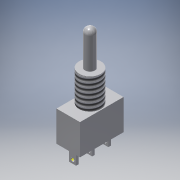
# Autodesk Inventor part: 1MS2
Saved by Autodesk Inventor 2016 (Build 200138000, 138)
## iProperties
Created: 2016-06-17
Part Number: 1MS2
Material: Aluminum
Document SubType Name: Modeling
Designer: Tyler
Density: 2.71 g/cm^3
Appearance: Satin
Author: Tyler
Autodesk Inventor part; units mm, degrees
ref_plane "YZ Plane" through (0, 0, 0) normal (1, 0, 0) x (0, 1, 0)
ref_plane "XZ Plane" through (0, 0, 0) normal (0, 1, 0) x (-1, 0, 0)
ref_plane "XY Plane" through (0, 0, 0) normal (0, 0, 1) x (1, 0, 0)
sketch "Sketch1" plane through (0, 0, 0) normal (0, 0, 1) x (1, 0, 0)
  line L0 (-3.43, -6.35) -> (3.43, -6.35)
  line L1 (3.43, -6.35) -> (3.43, 6.35)
  line L2 (3.43, 6.35) -> (-3.43, 6.35)
  line L3 (-3.43, 6.35) -> (-3.43, -6.35)
  line L4 (-3.43, -6.35) -> (3.43, 6.35) construction
  line L5 (3.43, -6.35) -> (-3.43, 6.35) construction
  point P0 (0, 0)
  dimension "d0" = 6.86
  dimension "d1" = 12.7
  constraints: 12 end point, 2 midpoint, 2 parallel, 1 horizontal, 1 perpendicular
  measures "d0" distance of L2.end L1.end
  measures "d1" distance of L1.end L0.end
extrude "Extrusion1" add sketch "Sketch1" against normal blind 8.89
sketch "Sketch2" plane through (0, 0, 0) normal (0, 0, 1) x (1, 0, 0)
  circle A0 centre (0, 0) radius 3.175
  dimension "d35" = 6.35
  constraints: 1 centre point, 1 coincident
  measures "d35" diameter of A0
extrude "Extrusion2" add sketch "Sketch2" along normal blind 8.89
sketch "Sketch3" plane through (0, 0, -8.89) normal (0, 0, -1) x (-1, 0, 0)
  line L0 (-1.015, -0.38) -> (1.015, -0.38)
  line L1 (1.015, -0.38) -> (1.015, 0.38)
  line L2 (1.015, 0.38) -> (-1.015, 0.38)
  line L3 (-1.015, 0.38) -> (-1.015, -0.38)
  line L4 (-1.015, -0.38) -> (1.015, 0.38) construction
  line L5 (1.015, -0.38) -> (-1.015, 0.38) construction
  line L6 (-1.015, -5.08) -> (1.015, -5.08)
  line L7 (1.015, -5.08) -> (1.015, -4.32)
  line L8 (1.015, -4.32) -> (-1.015, -4.32)
  line L9 (-1.015, -4.32) -> (-1.015, -5.08)
  line L10 (-1.015, -5.08) -> (1.015, -4.32) construction
  line L11 (1.015, -5.08) -> (-1.015, -4.32) construction
  line L12 (-1.015, -9.78) -> (1.015, -9.78) construction
  line L13 (1.015, -9.78) -> (1.015, -9.02) construction
  line L14 (1.015, -9.02) -> (-1.015, -9.02) construction
  line L15 (-1.015, -9.02) -> (-1.015, -9.78) construction
  line L16 (-1.015, -9.78) -> (1.015, -9.02) construction
  line L17 (1.015, -9.78) -> (-1.015, -9.02) construction
  line L18 (-1.015, 4.32) -> (1.015, 4.32)
  line L19 (1.015, 4.32) -> (1.015, 5.08)
  line L20 (1.015, 5.08) -> (-1.015, 5.08)
  line L21 (-1.015, 5.08) -> (-1.015, 4.32)
  line L22 (-1.015, 4.32) -> (1.015, 5.08) construction
  line L23 (1.015, 4.32) -> (-1.015, 5.08) construction
  point P0 (0, 0)
  point P1 (0, 4.7)
  dimension "d6" = 2.03
  dimension "d7" = 0.76
  dimension "d10" = 4.7
  dimension "d17" = 4.7
  constraints: 48 end point, 4 midpoint, 2 collinear, 2 parallel, 2 vertical, 1 horizontal, 1 perpendicular, 29 other
  measures "d6" distance of L2.end L1.end
  measures "d7" distance of L1.end L0.end
  measures "d10" distance of L0.start L6.start
  measures "d17" distance of L0.start L18.start
extrude "Extrusion3" add sketch "Sketch3" along normal blind 3.96
sketch "Sketch4" plane through (-1.015, 5.08, -8.89) normal (0, 1, 0) x (1, 0, 0)
  line L0 (2.03, 0) -> (2.03, 3.96) projected
  line L1 (0, 3.96) -> (2.03, 3.96) projected
  circle A0 centre (1.015, 2.96) radius 0.5
  point P0 (1.015, -8.89)
  dimension "d24" = 1
  dimension "d25" = 1
  dimension "d26" = 1.015
  constraints: 1 centre point
  measures "d24" diameter of A0
  measures "d25" distance from line of A0.centre L1
  measures "d26" distance from line of L0 A0.centre
extrude "Extrusion4" cut sketch "Sketch4" against normal through all
sketch "Sketch6" plane through (0, 0, 8.89) normal (0, 0, 1) x (1, 0, 0)
  circle A0 centre (0, 0) radius 1.46
  circle A1 centre (0, 0) radius 3.175 projected
  dimension "d29" = 2.92
  constraints: 1 centre point, 1 coincident
  measures "d29" diameter of A0
extrude "Extrusion5" add sketch "Sketch6" along normal blind 10.41 contours A0
fillet "Fillet1" radius 1.46 1 edges at (-1.46, 0, 19.3)
thread "Thread1" size "1/4-20 UNC" class "2A" standard "ANSI Unified Screw Threads" full length
sketch "Sketch7" plane through (-1.015, -5.08, -8.89) normal (0, -1, 0) x (1, 0, 0)
  circle A0 centre (1.015, -2.96) radius 0.5 projected
sketch "Sketch8" plane through (-1.015, -0.38, -8.89) normal (0, -1, 0) x (1, 0, 0)
  circle A0 centre (1.015, -2.96) radius 0.5 projected
sketch "Sketch9" plane through (-1.015, 4.32, -8.89) normal (0, -1, 0) x (1, 0, 0)
  circle A0 centre (1.015, -2.96) radius 0.5 projected
body "Solid1"
